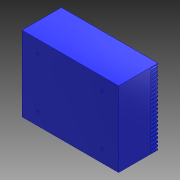
# Autodesk Inventor part: WR-LEN-base
Saved by Autodesk Inventor 2018 (Build 220112000, 112)
## iProperties
Created: 2022-04-20
Part Number: WR-LEN-base
Material: Generic
Document SubType Name: Modeling
Designer: pollak
Density: 1 g/cm^3
Appearance: Blue - Wall Paint - Glossy
Author: pollak
Autodesk Inventor part; units mm, degrees
ref_plane "YZ Plane" through (0, 0, 0) normal (1, 0, 0) x (0, 1, 0)
ref_plane "XZ Plane" through (0, 0, 0) normal (0, 1, 0) x (-1, 0, 0)
ref_plane "XY Plane" through (0, 0, 0) normal (0, 0, 1) x (1, 0, 0)
sketch "Sketch1" plane through (0, 0, 0) normal (0, 1, 0) x (-1, 0, 0)
  line L0 (67.5, 52.5) -> (-67.5, 52.5)
  line L1 (-67.5, 52.5) -> (-67.5, -52.5)
  line L2 (-67.5, -52.5) -> (67.5, -52.5)
  line L3 (67.5, -52.5) -> (67.5, 52.5)
  line L4 (67.5, 52.5) -> (-67.5, -52.5) construction
  line L5 (-67.5, 52.5) -> (67.5, -52.5) construction
  point P0 (0, 0)
  dimension "d0" = 135
  dimension "d1" = 105
  constraints: 12 end point, 2 midpoint, 2 parallel, 1 horizontal, 1 perpendicular
  measures "d0" distance of L2.end L1.end
  measures "d1" distance of L1.end L0.end
extrude "Extrusion1" add sketch "Sketch1" along normal blind 55
sketch "Sketch2" plane through (0, 55, 0) normal (0, 1, 0) x (1, 0, 0)
  line L0 (67.5, -52.5) -> (67.5, 52.5) projected
  line L1 (-67.5, -1.5) -> (67.5, -1.5)
  line L2 (67.5, -1.5) -> (67.5, 1.5)
  line L3 (67.5, 1.5) -> (-67.5, 1.5)
  line L4 (-67.5, 1.5) -> (-67.5, -1.5)
  line L5 (-67.5, -1.5) -> (67.5, 1.5) construction
  line L6 (67.5, -1.5) -> (-67.5, 1.5) construction
  line L7 (-67.5, 3.5) -> (67.5, 3.5)
  line L8 (67.5, 3.5) -> (67.5, 6.5)
  line L9 (67.5, 6.5) -> (-67.5, 6.5)
  line L10 (-67.5, 6.5) -> (-67.5, 3.5)
  line L11 (-67.5, 3.5) -> (67.5, 6.5) construction
  line L12 (67.5, 3.5) -> (-67.5, 6.5) construction
  line L13 (67.5, -3.5) -> (-67.5, -3.5)
  line L14 (-67.5, -3.5) -> (-67.5, -6.5)
  line L15 (-67.5, -6.5) -> (67.5, -6.5)
  line L16 (67.5, -6.5) -> (67.5, -3.5)
  line L17 (67.5, -8.5) -> (-67.5, -8.5)
  line L18 (-67.5, -8.5) -> (-67.5, -11.5)
  line L19 (-67.5, -11.5) -> (67.5, -11.5)
  line L20 (67.5, -11.5) -> (67.5, -8.5)
  line L21 (67.5, -13.5) -> (-67.5, -13.5)
  line L22 (-67.5, -13.5) -> (-67.5, -16.5)
  line L23 (-67.5, -16.5) -> (67.5, -16.5)
  line L24 (67.5, -16.5) -> (67.5, -13.5)
  line L25 (67.5, 11.5) -> (-67.5, 11.5)
  line L26 (-67.5, 11.5) -> (-67.5, 8.5)
  line L27 (-67.5, 8.5) -> (67.5, 8.5)
  line L28 (67.5, 8.5) -> (67.5, 11.5)
  line L29 (67.5, 13.5) -> (-67.5, 13.5)
  line L30 (-67.5, 13.5) -> (-67.5, 16.5)
  line L31 (-67.5, 16.5) -> (67.5, 16.5)
  line L32 (67.5, 16.5) -> (67.5, 13.5)
  line L33 (67.5, 23.5) -> (-67.5, 23.5)
  line L34 (-67.5, 23.5) -> (-67.5, 26.5)
  line L35 (-67.5, 26.5) -> (67.5, 26.5)
  line L36 (67.5, 26.5) -> (67.5, 23.5)
  line L37 (67.5, 18.5) -> (-67.5, 18.5)
  line L38 (-67.5, 18.5) -> (-67.5, 21.5)
  line L39 (-67.5, 21.5) -> (67.5, 21.5)
  line L40 (67.5, 21.5) -> (67.5, 18.5)
  line L41 (67.5, 28.5) -> (-67.5, 28.5)
  line L42 (-67.5, 28.5) -> (-67.5, 31.5)
  line L43 (-67.5, 31.5) -> (67.5, 31.5)
  line L44 (67.5, 31.5) -> (67.5, 28.5)
  line L45 (67.5, -41.5) -> (-67.5, -41.5)
  line L46 (-67.5, -41.5) -> (-67.5, -38.5)
  line L47 (-67.5, -38.5) -> (67.5, -38.5)
  line L48 (67.5, -38.5) -> (67.5, -41.5)
  line L49 (67.5, -36.5) -> (-67.5, -36.5)
  line L50 (-67.5, -36.5) -> (-67.5, -33.5)
  line L51 (-67.5, -33.5) -> (67.5, -33.5)
  line L52 (67.5, -33.5) -> (67.5, -36.5)
  line L53 (67.5, -31.5) -> (-67.5, -31.5)
  line L54 (-67.5, -31.5) -> (-67.5, -28.5)
  line L55 (-67.5, -28.5) -> (67.5, -28.5)
  line L56 (67.5, -28.5) -> (67.5, -31.5)
  line L57 (67.5, -26.5) -> (-67.5, -26.5)
  line L58 (-67.5, -26.5) -> (-67.5, -23.5)
  line L59 (-67.5, -23.5) -> (67.5, -23.5)
  line L60 (67.5, -23.5) -> (67.5, -26.5)
  line L61 (67.5, -21.5) -> (-67.5, -21.5)
  line L62 (-67.5, -21.5) -> (-67.5, -18.5)
  line L63 (-67.5, -18.5) -> (67.5, -18.5)
  line L64 (67.5, -18.5) -> (67.5, -21.5)
  line L65 (67.5, 33.5) -> (-67.5, 33.5)
  line L66 (-67.5, 33.5) -> (-67.5, 36.5)
  line L67 (-67.5, 36.5) -> (67.5, 36.5)
  line L68 (67.5, 36.5) -> (67.5, 33.5)
  line L69 (67.5, 38.5) -> (-67.5, 38.5)
  line L70 (-67.5, 38.5) -> (-67.5, 41.5)
  line L71 (-67.5, 41.5) -> (67.5, 41.5)
  line L72 (67.5, 41.5) -> (67.5, 38.5)
  line L73 (67.5, 43.5) -> (-67.5, 43.5)
  line L74 (-67.5, 43.5) -> (-67.5, 46.5)
  line L75 (-67.5, 46.5) -> (67.5, 46.5)
  line L76 (67.5, 46.5) -> (67.5, 43.5)
  line L77 (67.5, -43.5) -> (-67.5, -43.5)
  line L78 (-67.5, -43.5) -> (-67.5, -46.5)
  line L79 (-67.5, -46.5) -> (67.5, -46.5)
  line L80 (67.5, -46.5) -> (67.5, -43.5)
  line L81 (67.5, -48.5) -> (-67.5, -48.5)
  line L82 (-67.5, -48.5) -> (-67.5, -51.5)
  line L83 (-67.5, -51.5) -> (67.5, -51.5)
  line L84 (67.5, -51.5) -> (67.5, -48.5)
  line L85 (67.8672, 48.5) -> (-67.1328, 48.5)
  line L86 (-67.1328, 48.5) -> (-67.1328, 51.5)
  line L87 (-67.1328, 51.5) -> (67.8672, 51.5)
  line L88 (67.8672, 51.5) -> (67.8672, 48.5)
  point P0 (0, 0)
  point P1 (0, 5)
  dimension "d4" = 3
  dimension "d5" = 135
  dimension "d6" = 2
  dimension "d7" = 0
  dimension "d8" = 3
  dimension "d9" = 135
  dimension "d10" = 3
  dimension "d11" = 135
  dimension "d12" = 3
  dimension "d13" = 135
  dimension "d14" = 3
  dimension "d15" = 135
  dimension "d16" = 3
  dimension "d17" = 135
  dimension "d18" = 3
  dimension "d19" = 2
  dimension "d20" = 2
  dimension "d21" = 2
  dimension "d22" = 2
  dimension "d23" = 2
  dimension "d24" = 135
  dimension "d25" = 3
  dimension "d26" = 135
  dimension "d27" = 3
  dimension "d28" = 135
  dimension "d29" = 3
  dimension "d30" = 135
  dimension "d31" = 3
  dimension "d32" = 135
  dimension "d33" = 3
  dimension "d34" = 135
  dimension "d35" = 3
  dimension "d36" = 135
  dimension "d37" = 3
  dimension "d38" = 135
  dimension "d39" = 3
  dimension "d40" = 135
  dimension "d41" = 3
  dimension "d42" = 2
  dimension "d43" = 2
  dimension "d44" = 2
  dimension "d45" = 2
  dimension "d46" = 2
  dimension "d47" = 2
  dimension "d48" = 2
  dimension "d49" = 2
  dimension "d50" = 2
  dimension "d51" = 135
  dimension "d52" = 3
  dimension "d53" = 135
  dimension "d54" = 3
  dimension "d55" = 135
  dimension "d56" = 3
  dimension "d57" = 135
  dimension "d58" = 3
  dimension "d59" = 2
  dimension "d60" = 2
  dimension "d61" = 2
  dimension "d62" = 2
  dimension "d63" = 135
  dimension "d64" = 3
  dimension "d65" = 2
  constraints: 176 end point, 42 parallel, 21 horizontal, 21 perpendicular, 4 midpoint, 19 other
  measures "d4" distance of L2.end L1.end
  measures "d5" distance of L9.end L8.end
  measures "d6" distance between parallel lines of L7 L3
  measures "d7" horizontal extent of L8
  measures "d8" distance between parallel lines of L9 L7
  measures "d9" distance of L15.end L14.end
  measures "d10" distance of L14.end L13.end
  measures "d11" distance of L19.end L18.end
  measures "d12" distance of L18.end L17.end
  measures "d13" distance of L23.end L22.end
  measures "d14" distance of L22.end L21.end
  measures "d15" distance of L27.end L26.end
  measures "d16" distance of L26.end L25.end
  measures "d17" distance of L30.end L31.end
  measures "d18" distance of L29.end L30.end
  measures "d19" distance between parallel lines of L19 L21
  measures "d20" distance between parallel lines of L15 L17
  measures "d21" distance between parallel lines of L1 L13
  measures "d22" distance between parallel lines of L25 L29
  measures "d23" distance between parallel lines of L9 L27
  measures "d24" distance of L34.end L35.end
  measures "d25" distance of L33.end L34.end
  measures "d26" distance of L38.end L39.end
  measures "d27" distance of L37.end L38.end
  measures "d28" distance of L42.end L43.end
  measures "d29" distance of L41.end L42.end
  measures "d30" distance of L46.end L47.end
  measures "d31" distance of L45.end L46.end
  measures "d32" distance of L50.end L51.end
  measures "d33" distance of L49.end L50.end
  measures "d34" distance of L54.end L55.end
  measures "d35" distance of L53.end L54.end
  measures "d36" distance of L58.end L59.end
  measures "d37" distance of L57.end L58.end
  measures "d38" distance of L62.end L63.end
  measures "d39" distance of L61.end L62.end
  measures "d40" distance of L66.end L67.end
  measures "d41" distance of L65.end L66.end
  measures "d42" distance between parallel lines of L31 L37
  measures "d43" distance between parallel lines of L33 L39
  measures "d44" distance between parallel lines of L41 L35
  measures "d45" distance between parallel lines of L65 L43
  measures "d46" distance between parallel lines of L63 L23
  measures "d47" distance between parallel lines of L61 L59
  measures "d48" distance between parallel lines of L57 L55
  measures "d49" distance between parallel lines of L53 L51
  measures "d50" distance between parallel lines of L49 L47
  measures "d51" distance of L70.end L71.end
  measures "d52" distance of L69.end L70.end
  measures "d53" distance of L74.end L75.end
  measures "d54" distance of L73.end L74.end
  measures "d55" distance of L79.end L78.end
  measures "d56" distance of L78.end L77.end
  measures "d57" distance of L83.end L82.end
  measures "d58" distance of L82.end L81.end
  measures "d59" distance between parallel lines of L45 L77
  measures "d60" distance between parallel lines of L79 L81
  measures "d61" distance between parallel lines of L67 L69
  measures "d62" distance between parallel lines of L73 L71
  measures "d63" distance of L86.end L87.end
  measures "d64" distance of L85.end L86.end
  measures "d65" distance between parallel lines of L85 L75
extrude "Extrusion2" cut sketch "Sketch2" against normal blind 10
sketch "Sketch3" plane through (0, 0, 0) normal (0, -1, 0) x (1, 0, 0)
  line L0 (45, 35) -> (-45, 35) construction
  line L1 (-45, 35) -> (-45, -35) construction
  line L2 (-45, -35) -> (45, -35) construction
  line L3 (45, -35) -> (45, 35) construction
  line L4 (45, 35) -> (-45, -35) construction
  line L5 (-45, 35) -> (45, -35) construction
  point P0 (0, 0)
  dimension "d68" = 90
  dimension "d69" = 70
  constraints: 12 end point, 4 coincident, 2 midpoint, 2 parallel, 1 horizontal, 1 perpendicular
  measures "d68" distance of L2.end L1.end
  measures "d69" distance of L1.end L0.end
hole "Hole1" at (45, 0, -35) at (-45, 0, -35) at (-45, 0, 35) at (45, 0, 35) direction (0, 1, 0) diameter 3.4 depth 8 tip angle 118
body "Solid1"
